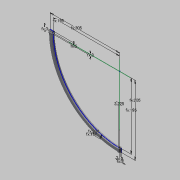
# Autodesk Inventor part: ArcFrameRa
Saved by Autodesk Inventor 2015 (Build 190159000, 159)
## iProperties
Created: 2016-06-12
Part Number: ArcFrameRa
Material: 一般
Document SubType Name: Modeling
Designer: kumagai
Density: 1 g/cm^3
Appearance: 既定
Author: kumagai
Autodesk Inventor part; units mm, degrees
ref_plane "YZ Plane" through (0, 0, 0) normal (1, 0, 0) x (0, 1, 0)
ref_plane "XZ Plane" through (0, 0, 0) normal (0, 1, 0) x (-1, 0, 0)
ref_plane "XY Plane" through (0, 0, 0) normal (0, 0, 1) x (1, 0, 0)
sketch "スケッチ1" plane through (0, 0, 0) normal (0, 1, 0) x (-1, 0, 0)
  line L0 (0, -149.7212) -> (0, 30.7869) projected
  line L1 (-30.7969, 0) -> (149.7814, 0) projected
  arc A0 (3.2253, -195.9735) -> (195.977, -3) centre (0, 0) ccw
  arc A1 (3.2253, -203.9745) -> (203.9779, -3) centre (0, 0) ccw
  line L2 (195, 3) -> (195, 5)
  line L3 (195, 5) -> (205, 5)
  line L4 (205, 5) -> (205, 3)
  line L5 (205, 3) -> (195, 3)
  line L6 (203.9779, -3) -> (195.977, -3)
  line L7 (-3, -195) -> (-5, -195)
  line L8 (-5, -195) -> (-5, -205)
  line L9 (-5, -205) -> (-3, -205)
  line L10 (-3, -205) -> (-3, -195)
  line L11 (3.2253, -195.9735) -> (3.2253, -203.9745)
  dimension "d0" = 204
  dimension "d1" = 196
  dimension "d2" = 205
  dimension "d3" = 195
  dimension "d4" = 5
  dimension "d5" = 3
  dimension "d6" = 195
  dimension "d7" = 205
  dimension "d8" = 5
  dimension "d9" = 3
  dimension "d14" = 3
  dimension "d15" = 3.2253
  constraints: 20 end point, 5 parallel, 4 point on circle, 2 centre point, 2 coincident, 2 horizontal, 1 perpendicular
  measures "d0" radius of A1
  measures "d1" radius of A0
  measures "d2" distance between parallel lines of L4 L0
  measures "d3" distance between parallel lines of L0 L2
  measures "d4" distance between parallel lines of L3 L1
  measures "d5" distance between parallel lines of L1 L5
  measures "d6" distance between parallel lines of L1 L7
  measures "d7" distance between parallel lines of L1 L9
  measures "d8" distance between parallel lines of L0 L8
  measures "d9" distance between parallel lines of L0 L10
  measures "d14" distance between parallel lines of L6 L1
  measures "d15" distance between parallel lines of L0 L11
extrude "押し出し1" add sketch "スケッチ1" along normal mid plane 8 contours A0 L6 A1 L11
revolve "回転1" add sketch "スケッチ1" angle 360 about axis through (0, 0, 0) along (-1, 0, 0) contours L2 L3 L4 L5
revolve "回転2" add sketch "スケッチ1" angle 360 about axis through (0, 0, 0) along (0, 0, 1) contours L10 L9 L8 L7
equation "\"d0\" = FrameRadius + 0.5 * FrameThickness"
equation "\"d1\" = FrameRadius - 0.5 * FrameThickness"
equation "\"d2\" = FrameRadius + 0.5 * BossLength"
equation "\"d3\" = FrameRadius - 0.5 * BossLength"
equation "\"d4\" = BossRadius"
equation "\"d5\" = BossHoleRadius"
equation "\"d6\" = FrameRadius - 0.5 * BossLength"
equation "\"d7\" = FrameRadius + 0.5 * BossLength"
equation "\"d8\" = BossRadius"
equation "\"d9\" = BossHoleRadius"
equation "\"d14\" = BossHoleRadius"
equation "\"d10\" = FrameThickness"
equation "\"FrameThickness\" = 8"
equation "\"BossRadius\" = 5"
equation "\"BossHoleRadius\" = 3"
equation "\"FrameRadius\" = 200"
equation "\"BossLength\" = 10"
